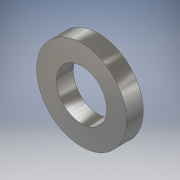
# Autodesk Inventor part: 1-4inch_BearingSpacer_Piece1
Saved by Autodesk Inventor 2018 (Build 220112000, 112)
## iProperties
Created: 2018-01-21
Part Number: 1-4inch_BearingSpacer_Piece1
Material: Generic
Document SubType Name: Modeling
Designer: Olivier
Density: 1 g/cm^3
Appearance: Default
Author: Olivier
Autodesk Inventor part; units mm, degrees
ref_plane "YZ Plane" through (0, 0, 0) normal (1, 0, 0) x (0, 1, 0)
ref_plane "XZ Plane" through (0, 0, 0) normal (0, 1, 0) x (-1, 0, 0)
ref_plane "XY Plane" through (0, 0, 0) normal (0, 0, 1) x (1, 0, 0)
sketch "Sketch1" plane through (0, 0, 0) normal (0, 0, 1) x (1, 0, 0)
  circle A0 centre (0, 0) radius 17
  circle A1 centre (0, 0) radius 17
  circle A2 centre (0, 0) radius 9.525
  dimension "d4" = 19.05
  constraints: 3 centre point, 1 coincident
  measures "d4" diameter of A2
extrude "Extrusion2" add sketch "Sketch1" along normal blind 6.35
body "Solid2"
